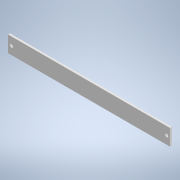
# Autodesk Inventor part: Base_Carril
Saved by Autodesk Inventor 2022 (Build 260153000, 153)
## iProperties
Created: 2022-01-30
Part Number: Base_Carril
Material: Generic
Document SubType Name: Modeling
Designer: katha
Density: 1 g/cm^3
Appearance: Default
Author: katha
Autodesk Inventor part; units mm, degrees
ref_plane "YZ Plane" through (0, 0, 0) normal (1, 0, 0) x (0, 1, 0)
ref_plane "XZ Plane" through (0, 0, 0) normal (0, 1, 0) x (-1, 0, 0)
ref_plane "XY Plane" through (0, 0, 0) normal (0, 0, 1) x (1, 0, 0)
sketch "Sketch1" plane through (0, 0, 0) normal (0, 0, 1) x (1, 0, 0)
  line L0 (-125, 12.5) -> (125, 12.5)
  line L1 (125, 12.5) -> (125, -12.5)
  line L2 (125, -12.5) -> (-125, -12.5)
  line L3 (-125, -12.5) -> (-125, 12.5)
  line L4 (-125, 12.5) -> (125, -12.5) construction
  line L5 (125, 12.5) -> (-125, -12.5) construction
  point P0 (0, 0)
  dimension "d0" = 250
  dimension "d1" = 25
  constraints: 12 end point, 2 midpoint, 2 parallel, 1 horizontal, 1 perpendicular
  measures "d0" distance of L1.end L2.end
  measures "d1" distance of L0.end L1.end
extrude "Extrusion1" add sketch "Sketch1" along normal blind 3
sketch "Sketch2" plane through (0, 0, 0) normal (0, 0, -1) x (-1, 0, 0)
  circle A0 centre (-120, 0) radius 2.5 projected
  circle A1 centre (-120, 0) radius 2.5
  line L0 (0, 0) -> (0, -18.9534) construction
  circle A2 centre (120, 0) radius 2.5
  constraints: 2 centre point, 2 end point, 1 coincident, 1 concentric, 1 symmetric about line, 1 vertical, 1 other
extrude "Extrusion2" cut sketch "Sketch2" against normal blind 3
body "Solid1"
